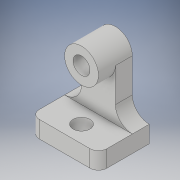
# Autodesk Inventor part: Part8
Saved by Autodesk Inventor 2017 (Build 210142000, 142)
## iProperties
Created: 2016-11-03
Part Number: Part8
Material: Generic
Document SubType Name: Modeling
Designer: s411888
Density: 1 g/cm^3
Appearance: Default
Author: s411888
Autodesk Inventor part; units mm, degrees
ref_plane "YZ Plane" through (0, 0, 0) normal (1, 0, 0) x (0, 1, 0)
ref_plane "XZ Plane" through (0, 0, 0) normal (0, 1, 0) x (-1, 0, 0)
ref_plane "XY Plane" through (0, 0, 0) normal (0, 0, 1) x (1, 0, 0)
sketch "Sketch1" plane through (0, 0, 0) normal (0, 1, 0) x (-1, 0, 0)
  line L0 (28.0719, 23.0631) -> (-22.7281, 23.0631)
  line L1 (-22.7281, 23.0631) -> (-22.7281, -15.0369)
  line L2 (-22.7281, -15.0369) -> (28.0719, -15.0369)
  line L3 (28.0719, -15.0369) -> (28.0719, 23.0631)
  point P0 (0, 0)
  dimension "d0" = 50.8
  dimension "d1" = 38.1
  constraints: 8 end point, 2 parallel, 1 horizontal, 1 perpendicular
  measures "d0" distance of L2.end L1.end
  measures "d1" distance of L1.end L0.end
extrude "Extrusion1" add sketch "Sketch1" along normal blind 12.7
sketch "Sketch2" plane through (0, 12.7, 0) normal (0, 1, 0) x (1, 0, 0)
  line L0 (22.7281, -23.0631) -> (22.7281, 15.0369) projected
  line L1 (22.7281, 15.0369) -> (10.0281, 15.0369)
  line L2 (10.0281, 15.0369) -> (10.0281, 2.3369)
  line L3 (10.0281, 2.3369) -> (22.7281, 2.3369)
  line L4 (22.7281, 2.3369) -> (22.7281, 15.0369)
  line L5 (22.7281, 15.0369) -> (-28.0719, 15.0369) projected
  line L6 (-28.0719, 15.0369) -> (-15.3719, 15.0369)
  line L7 (-15.3719, 15.0369) -> (-15.3719, 2.3369)
  line L8 (-15.3719, 2.3369) -> (-28.0719, 2.3369)
  line L9 (-28.0719, 2.3369) -> (-28.0719, 15.0369)
  line L10 (-15.3719, 15.0369) -> (10.0281, 15.0369)
  line L11 (10.0281, 15.0369) -> (10.0281, 2.3369)
  line L12 (10.0281, 2.3369) -> (-15.3719, 2.3369)
  line L13 (-15.3719, 2.3369) -> (-15.3719, 15.0369)
  point P0 (0, 0)
  dimension "d4" = 12.7
  dimension "d5" = 12.7
  dimension "d6" = 12.7
  dimension "d7" = 12.7
  constraints: 24 end point, 6 parallel, 3 horizontal, 3 perpendicular
  measures "d4" distance of L3.end L2.end
  measures "d5" distance of L2.end L1.end
  measures "d6" distance of L7.end L8.end
  measures "d7" distance of L6.end L7.end
extrude "Extrusion2" add sketch "Sketch2" along normal blind 38.1 contours L12 L7 L5 L2
fillet "Fillet1" radius 12.7 1 edges at (10.0281, 12.7, -8.6869)
fillet "Fillet2" radius 12.7 1 edges at (-15.3719, 12.7, -8.6869)
sketch "Sketch3" plane through (22.7281, 0, -15.0369) normal (0, 0, -1) x (-1, 0, 0)
  line L0 (12.7, 25.4) -> (12.7, 50.8) projected
  line L1 (12.7, 50.8) -> (25.4, 50.8)
  line L2 (12.7, 50.8) -> (38.1, 50.8) projected
  circle A0 centre (25.4, 50.8) radius 12.7
  point P0 (22.7281, 0)
  dimension "d12" = 12.7
  dimension "d13" = 25.4
  constraints: 2 end point, 1 centre point, 1 coincident, 1 midpoint
  measures "d12" distance of L0.end L1.end
  measures "d13" diameter of A0
extrude "Extrusion3" add sketch "Sketch3" against normal blind 25.4
sketch "Sketch4" plane through (-2.6719, 50.8, 10.3631) normal (0, 0, 1) x (1, 0, 0)
  circle A0 centre (0, 0) radius 6.35
  point P0 (2.6719, -50.8)
  dimension "d16" = 12.7
  constraints: 1 centre point
  measures "d16" diameter of A0
extrude "Extrusion4" cut sketch "Sketch4" against normal blind 25.4
fillet "Fillet3" radius 6.35 1 edges at (22.7281, 6.35, 23.0631)
fillet "Fillet4" radius 6.35 1 edges at (-28.0719, 6.35, 23.0631)
sketch "Sketch6" plane through (0, 12.7, 0) normal (0, 1, 0) x (1, 0, 0)
  line L0 (-21.7219, -23.0631) -> (16.3781, -23.0631) projected
  line L1 (-2.6719, -23.0631) -> (-2.6719, -10.3631)
  circle A0 centre (-2.6719, -10.3631) radius 6.35
  point P0 (0, 0)
  dimension "d22" = 12.7
  dimension "d23" = 12.7
  constraints: 2 end point, 1 centre point, 1 coincident, 1 midpoint, 1 vertical
  measures "d22" distance of L1.start L1.end
  measures "d23" diameter of A0
extrude "Extrusion5" cut sketch "Sketch6" against normal blind 25.4
body "Solid1"
